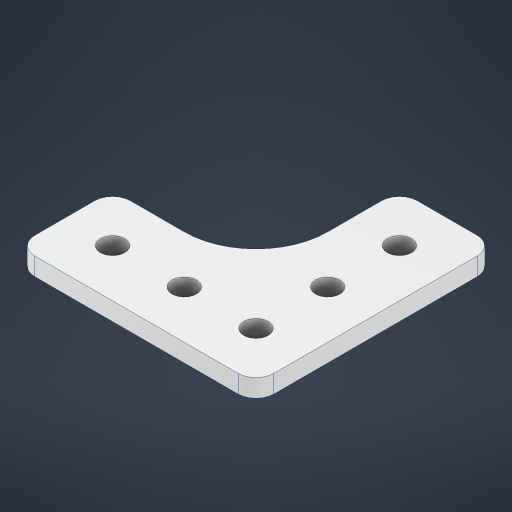
# Autodesk Inventor part: STRU_009_FrameBracket_90
Saved by Autodesk Inventor 2024.2 (Build 282272000, 272)
## iProperties
Created: 2024-07-24
Part Number: STRU_009_FrameBracket_90
Material: Aluminum 6061
Document SubType Name: Modeling
Designer: Bryan
Density: 2.7 g/cm^3
Appearance: Aluminum - Flat
Mass: 31.7373 g
Surface Area: 65.4479 cm^2
Volume: 11.7545 cm^3
Author: Bryan
Autodesk Inventor part; units mm, degrees
ref_plane "YZ Plane" through (0, 0, 0) normal (1, 0, 0) x (0, 1, 0)
ref_plane "XZ Plane" through (0, 0, 0) normal (0, 1, 0) x (-1, 0, 0)
ref_plane "XY Plane" through (0, 0, 0) normal (0, 0, 1) x (1, 0, 0)
sketch "Sketch1" plane through (0, 0, 0) normal (0, 1, 0) x (-1, 0, 0)
  line L0 (0, 0) -> (63.5, 0)
  line L1 (63.5, 0) -> (63.5, -25.4)
  line L2 (63.5, -25.4) -> (25.4, -25.4)
  line L3 (25.4, -25.4) -> (25.4, -63.5)
  line L4 (25.4, -63.5) -> (0, -63.5)
  line L5 (0, -63.5) -> (0, 0)
  circle A0 centre (12.7, -12.7) radius 3.2512
  line L6 (0, 0) -> (25.4, -25.4) construction
  circle A1 centre (31.75, -12.7) radius 3.2512
  circle A2 centre (50.8, -12.7) radius 3.2512
  circle A3 centre (12.7, -31.75) radius 3.2512
  circle A4 centre (12.7, -50.8) radius 3.2512
  point P0 (12.7, -12.7)
  dimension "d0" = 25.4
  dimension "d1" = 6.5024
  dimension "d2" = 19.05
  dimension "d3" = 19.05
  dimension "d4" = 12.7
  constraints: 14 end point, 7 perpendicular, 5 centre point, 4 equal radius, 2 horizontal alignment, 2 vertical alignment, 1 coincident, 1 horizontal, 1 midpoint, 2 other
  measures "d0" distance of L0.end L1.end
  measures "d1" diameter of A0
  measures "d2" distance of A0.centre A1.centre
  measures "d3" distance of A1.centre A2.centre
  measures "d4" distance from line of L1 A2.centre
extrude "Extrusion1" add sketch "Sketch1" along normal blind 4.7625
fillet "Fillet1" radius 4.7625 5 edges at (0, 2.3813, 0) (-63.5, 2.3813, 0) (-63.5, 2.3813, -25.4) (0, 2.3813, -63.5) (-25.4, 2.3813, -63.5)
fillet "Fillet2" radius 19.05 1 edges at (-25.4, 2.3813, -25.4)
body "Solid1"
